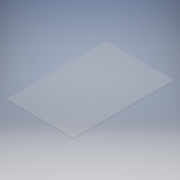
# Autodesk Inventor part: ElectricalBoard.ver1-1111-2019
Saved by Autodesk Inventor 2018 (Build 220112000, 112)
## iProperties
Created: 2019-11-12
Part Number: ElectricalBoard.ver1-1111-2019
Material: Polycarbonate, Clear
Document SubType Name: Modeling
Designer: JMHal
Density: 1.2 g/cm^3
Appearance: Polycarbonate - Clear
Author: JMHal
Autodesk Inventor part; units mm, degrees
ref_plane "YZ Plane" through (0, 0, 0) normal (1, 0, 0) x (0, 1, 0)
ref_plane "XZ Plane" through (0, 0, 0) normal (0, 1, 0) x (-1, 0, 0)
ref_plane "XY Plane" through (0, 0, 0) normal (0, 0, 1) x (1, 0, 0)
sketch "Sketch1" plane through (0, 0, 0) normal (0, 1, 0) x (-1, 0, 0)
  line L0 (0, 0) -> (393.7, 0)
  line L1 (393.7, 0) -> (393.7, -558.8)
  line L2 (393.7, -558.8) -> (0, -558.8)
  line L3 (0, -558.8) -> (0, 0)
  dimension "d0" = 393.7
  dimension "d1" = 558.8
  constraints: 8 end point, 2 parallel, 1 horizontal, 1 perpendicular
  measures "d0" distance of L1.end L2.end
  measures "d1" distance of L0.end L1.end
extrude "Extrusion1" add sketch "Sketch1" along normal blind 3.175
sketch "Sketch3" plane through (0, 3.175, 0) normal (0, 1, 0) x (1, 0, 0)
  line L0 (0, 0) -> (0, 558.8) projected
  line L1 (0, 327.1063) -> (0, 139.7813)
  line L2 (-393.7, 558.8) -> (-393.7, 0) projected
  line L3 (-393.7, 373.0625) -> (-190.5, 373.0625)
  line L4 (-190.5, 373.0625) -> (-190.5, 185.7375)
  line L5 (-190.5, 185.7375) -> (-393.7, 185.7375)
  line L6 (-393.7, 185.7375) -> (-393.7, 373.0625)
  point P0 (-190.5, 279.4)
  point P1 (-393.7, 279.4)
  dimension "d8" = 187.325
  dimension "d9" = 203.2
  constraints: 10 end point, 2 midpoint, 2 parallel, 2 point on line, 1 horizontal, 1 horizontal alignment, 1 perpendicular
  measures "d8" distance of L3.end L4.end
  measures "d9" distance of L3.start L3.end
extrude "Extrusion3" cut sketch "Sketch3" against normal up to surface (3.175 mm away)
body "Solid1"
